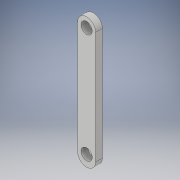
# Autodesk Inventor part: drawing bot arm
Saved by Autodesk Inventor 2019 (Build 230136000, 136)
## iProperties
Created: 2020-02-10
Part Number: drawing bot arm
Material: Generic
Document SubType Name: Modeling
Designer: user
Density: 1 g/cm^3
Appearance: Default
Author: user
Autodesk Inventor part; units mm, degrees
ref_plane "YZ Plane" through (0, 0, 0) normal (1, 0, 0) x (0, 1, 0)
ref_plane "XZ Plane" through (0, 0, 0) normal (0, 1, 0) x (-1, 0, 0)
ref_plane "XY Plane" through (0, 0, 0) normal (0, 0, 1) x (1, 0, 0)
sketch "Sketch1" plane through (0, 0, 0) normal (0, 0, 1) x (1, 0, 0)
  line L0 (-69.598, 209.799) -> (-69.598, -40.201) construction
  line L1 (-89.598, 209.799) -> (-89.598, -40.201)
  line L2 (-49.598, -40.201) -> (-49.598, 209.799)
  arc A0 (-49.598, 209.799) -> (-89.598, 209.799) centre (-69.598, 209.799) ccw
  arc A1 (-89.598, -40.201) -> (-49.598, -40.201) centre (-69.598, -40.201) ccw
  point P0 (0, 0)
  point P1 (-69.598, 84.799)
  dimension "d0" = 250
  dimension "d1" = 20
  constraints: 8 end point, 4 point on circle, 4 tangent, 2 centre point, 1 midpoint, 1 parallel, 1 vertical
  measures "d0" distance of L2.start L2.end
  measures "d1" radius of A1
extrude "Extrusion1" add sketch "Sketch1" along normal blind 15
sketch "Sketch2" plane through (0, 0, 0) normal (0, 0, -1) x (-1, 0, 0)
  line L0 (49.598, -40.201) -> (49.598, 209.799) projected
  circle A0 centre (69.598, 208.3571) radius 12.5
  point P0 (0, 0)
  point P1 (69.598, 88.3571)
  dimension "d4" = 20
  dimension "d5" = 25
  dimension "d6" = 120
  constraints: 1 centre point
  measures "d4" distance from line of L0 point (69.598, 88.357)
  measures "d5" diameter of A0
  measures "d6" distance of point (69.598, 88.357) A0.centre
extrude "Extrusion2" cut sketch "Sketch2" against normal blind 20
sketch "Sketch3" plane through (0, 0, 0) normal (0, 0, -1) x (-1, 0, 0)
  line L0 (89.598, 209.799) -> (89.598, -40.201) projected
  circle A0 centre (69.598, -35.201) radius 12.5
  point P0 (0, 0)
  point P1 (69.598, 84.799)
  dimension "d9" = 20
  dimension "d10" = 125
  dimension "d11" = 25
  dimension "d12" = 120
  dimension "d13" = 20
  constraints: 1 centre point
  measures "d9" distance from line of L0 point (69.598, 84.799)
  measures "d10" vertical distance of L0.end point (69.598, 84.799)
  measures "d11" diameter of A0
  measures "d12" distance of A0.centre point (69.598, 84.799)
  measures "d13" distance from line of A0.centre L0
extrude "Extrusion3" cut sketch "Sketch3" against normal blind 20
body "Solid1"
